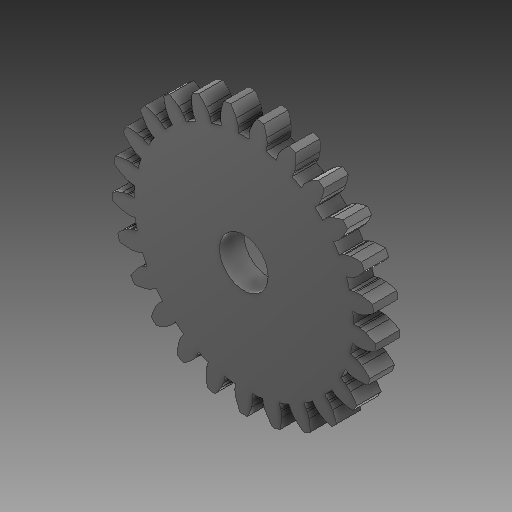
# Autodesk Inventor part: 歯車m2.z25
Saved by Autodesk Inventor 2020 (Build 240168000, 168)
## iProperties
Created: 2019-09-03
Part Number: 歯車m2.z25
Material: アセタール樹脂、黒
Document SubType Name: Modeling
Designer: 雪村
Density: 1.425 g/cm^3
Appearance: 滑らか - 黒
Mass: 7.88044 g
Surface Area: 64.9831 cm^2
Volume: 5.53013 cm^3
Description: ジュラコン 5t
Author: 雪村
Autodesk Inventor part; units mm, degrees
ref_plane "YZ Plane" through (0, 0, 0) normal (1, 0, 0) x (0, 1, 0)
ref_plane "XZ Plane" through (0, 0, 0) normal (0, 1, 0) x (-1, 0, 0)
ref_plane "XY Plane" through (0, 0, 0) normal (0, 0, 1) x (1, 0, 0)
sketch "スケッチ1" plane through (0, 0, 0) normal (0, 0, 1) x (1, 0, 0)
  arc A0 (1.1831, 23.814) -> (1.1255, 23.4653) centre (3.4046, 23.2682) ccw
  arc A1 (1.549, 24.9027) -> (1.1831, 23.814) centre (7.3031, 22.3628) ccw
  arc A2 (2.6687, 26.8678) -> (1.549, 24.9027) centre (11.5034, 20.532) ccw
  arc A3 (-4.7764, 23.36) -> (-4.7455, 23.008) centre (-2.4889, 23.3838) ccw
  arc A4 (-4.6927, 24.5056) -> (-4.7764, 23.36) centre (1.5122, 23.4765) ccw
  arc A5 (-4.0969, 26.6874) -> (-4.6927, 24.5056) centre (6.036, 22.7477) ccw
  arc A6 (-10.4358, 21.4383) -> (-10.3182, 21.105) centre (-8.226, 22.0302) ccw
  arc A7 (-10.6396, 22.5687) -> (-10.4358, 21.4383) centre (-4.3736, 23.115) ccw
  arc A8 (-10.605, 24.8301) -> (-10.6396, 22.5687) centre (0.1892, 23.5341) ccw
  arc A9 (-15.4394, 18.1695) -> (-15.2427, 17.876) centre (-13.4463, 19.2924) ccw
  arc A10 (-15.9179, 19.2137) -> (-15.4394, 18.1695) centre (-9.9847, 21.3011) ccw
  arc A11 (-16.4468, 21.4126) -> (-15.9179, 19.2137) centre (-5.6694, 22.8418) ccw
  arc A12 (-19.4729, 13.7591) -> (-19.2094, 13.5236) centre (-17.8217, 15.3423) ccw
  arc A13 (-20.1961, 14.6514) -> (-19.4729, 13.7591) centre (-14.9684, 18.1488) ccw
  arc A14 (-21.2552, 16.6498) -> (-20.1961, 14.6514) centre (-11.1719, 20.7143) ccw
  arc A15 (-22.2829, 8.4841) -> (-21.9691, 8.3216) centre (-21.0772, 10.4282) ccw
  arc A16 (-23.2052, 9.1685) -> (-22.2829, 8.4841) centre (-19.0115, 13.8562) ccw
  arc A17 (-24.7281, 10.8407) -> (-23.2052, 9.1685) centre (-15.9723, 17.2852) ccw
  arc A18 (-23.6927, 2.676) -> (-23.3484, 2.5967) centre (-23.0085, 4.8589) ccw
  arc A19 (-24.7563, 3.1096) -> (-23.6927, 2.676) centre (-21.8601, 8.6929) ccw
  arc A20 (-26.6472, 4.3505) -> (-24.7563, 3.1096) centre (-19.7691, 12.77) ccw
  arc A21 (-23.6139, -3.3002) -> (-23.2606, -3.2914) centre (-23.494, -1.0157) ccw
  arc A22 (-24.7519, -3.1447) -> (-23.6139, -3.3002) centre (-23.3352, 2.9834) ccw
  arc A23 (-26.892, -2.4131) -> (-24.7519, -3.1447) centre (-22.3238, 7.4524) ccw
  arc A24 (-22.0513, -9.069) -> (-21.7113, -8.9727) centre (-22.5033, -6.8265) ccw
  arc A25 (-23.1922, -9.2015) -> (-22.0513, -9.069) centre (-23.344, -2.9136) ccw
  arc A26 (-25.447, -9.025) -> (-23.1922, -9.2015) centre (-23.4758, 1.6665) ccw
  arc A27 (-19.1031, -14.268) -> (-18.7978, -14.0902) centre (-20.0986, -12.2084) ccw
  arc A28 (-20.1752, -14.6801) -> (-19.1031, -14.268) centre (-21.886, -8.6275) ccw
  arc A29 (-22.4031, -15.0699) -> (-20.1752, -14.6801) centre (-23.1527, -4.224) ccw
  arc A30 (-14.9546, -18.5705) -> (-14.7031, -18.3223) centre (-16.4311, -16.8231) ccw
  arc A31 (-15.8906, -19.2363) -> (-14.9546, -18.5705) centre (-19.0529, -13.7993) ccw
  arc A32 (-17.9515, -20.1679) -> (-15.8906, -19.2363) centre (-21.3749, -9.8492) ccw
  arc A33 (-9.8665, -21.7062) -> (-9.6846, -21.4032) centre (-11.7311, -20.3809) ccw
  arc A34 (-10.6075, -22.5837) -> (-9.8665, -21.7062) centre (-15.0226, -18.104) ccw
  arc A35 (-12.372, -23.9986) -> (-10.6075, -22.5837) centre (-18.254, -14.8554) ccw
  arc A36 (-4.1584, -23.4779) -> (-4.0576, -23.1392) centre (-6.294, -22.658) ccw
  arc A37 (-4.6579, -24.5122) -> (-4.1584, -23.4779) centre (-10.0483, -21.2712) ccw
  arc A38 (-6.0151, -26.3214) -> (-4.6579, -24.5122) centre (-13.9861, -18.9283) ccw
  arc A39 (1.811, -23.7745) -> (1.8244, -23.4214) centre (-0.4615, -23.5114) ccw
  arc A40 (1.5844, -24.9005) -> (1.811, -23.7745) centre (-4.4427, -23.1018) ccw
  arc A41 (0.7197, -26.9904) -> (1.5844, -24.9005) centre (-8.8394, -21.8118) ccw
  arc A42 (7.6665, -22.5772) -> (7.5917, -22.2318) centre (5.4, -22.8875) ccw
  arc A43 (7.7271, -23.7242) -> (7.6665, -22.5772) centre (1.4421, -23.4809) ccw
  arc A44 (7.4094, -25.9635) -> (7.7271, -23.7242) centre (-3.1373, -23.3248) ccw
  arc A45 (13.0404, -19.9613) -> (12.882, -19.6454) centre (10.9223, -20.8255) ccw
  arc A46 (13.3843, -21.0572) -> (13.0404, -19.9613) centre (7.2362, -22.3846) ccw
  arc A47 (13.6334, -23.3051) -> (13.3843, -21.0572) centre (2.7619, -23.3723) ccw
  arc A48 (17.5949, -16.0912) -> (17.3629, -15.8246) centre (15.7582, -17.455) ccw
  arc A49 (18.2005, -17.0671) -> (17.5949, -16.0912) centre (12.5757, -19.8817) ccw
  arc A50 (19.0009, -19.1825) -> (18.2005, -17.0671) centre (8.4876, -21.9511) ccw
  arc A51 (21.0438, -11.21) -> (20.7529, -11.0094) centre (19.604, -12.9877) ccw
  arc A52 (21.8731, -12.0046) -> (21.0438, -11.21) centre (17.125, -16.1297) ccw
  arc A53 (23.1744, -13.8545) -> (21.8731, -12.0046) centre (13.68, -19.1507) ccw
  arc A54 (23.1705, -5.6244) -> (22.8388, -5.5025) centre (22.2181, -7.7043) ccw
  arc A55 (24.1714, -6.1879) -> (23.1705, -5.6244) centre (20.5983, -11.3641) ccw
  arc A56 (25.8918, -7.656) -> (24.1714, -6.1879) centre (18.0128, -15.147) ccw
  arc A57 (23.8413, 0.3146) -> (23.4897, 0.3501) centre (23.436, -1.9369) ccw
  arc A58 (24.9508, 0.0177) -> (23.8413, 0.3146) centre (22.7773, -5.8845) ccw
  arc A59 (26.9823, -0.9764) -> (24.9508, 0.0177) centre (21.2138, -10.1915) ccw
  arc A60 (23.014, 6.2338) -> (22.6647, 6.1808) centre (23.1814, 3.9523) ccw
  arc A61 (24.1626, 6.2222) -> (23.014, 6.2338) centre (23.5251, -0.0352) ccw
  arc A62 (26.3775, 5.7645) -> (24.1626, 6.2222) centre (23.0818, -4.5957) ccw
  arc A63 (20.7407, 11.7613) -> (20.4155, 11.6231) centre (21.4702, 9.5931) ccw
  arc A64 (21.8561, 12.0357) -> (20.7407, 11.7613) centre (22.7948, 5.8164) ccw
  arc A65 (24.1152, 12.1432) -> (21.8561, 12.0357) centre (23.4996, 1.2889) ccw
  arc A66 (17.1642, 16.5498) -> (16.8836, 16.335) centre (18.41, 14.6311) ccw
  arc A67 (18.1763, 17.0929) -> (17.1642, 16.5498) centre (20.6321, 11.3025) ccw
  arc A68 (20.3377, 17.7589) -> (18.1763, 17.0929) centre (22.4408, 7.0925) ccw
  arc A69 (12.5092, 20.2984) -> (12.2908, 20.0206) centre (14.193, 18.7499) ccw
  arc A70 (13.3544, 21.0762) -> (12.5092, 20.2984) centre (17.1731, 16.0784) ccw
  arc A71 (15.2823, 22.2587) -> (13.3544, 21.0762) centre (19.9719, 12.4505) ccw
  arc A72 (7.0682, 22.7716) -> (6.9257, 22.4482) centre (9.0842, 21.6904) ccw
  arc A73 (7.6934, 23.7351) -> (7.0682, 22.7716) centre (12.6351, 19.8441) ccw
  arc A74 (9.2666, 25.36) -> (7.6934, 23.7351) centre (16.2481, 17.0261) ccw
  arc A75 (-1.1255, 23.4653) -> (-1.1831, 23.814) centre (-3.4046, 23.2682) ccw
  arc A76 (-1.1831, 23.814) -> (-1.549, 24.9027) centre (-7.3031, 22.3628) ccw
  arc A77 (-1.549, 24.9027) -> (-2.6687, 26.8678) centre (-11.5034, 20.532) ccw
  arc A78 (-6.9257, 22.4482) -> (-7.0682, 22.7716) centre (-9.0842, 21.6904) ccw
  arc A79 (-7.0682, 22.7716) -> (-7.6934, 23.7351) centre (-12.6351, 19.8441) ccw
  arc A80 (-7.6934, 23.7351) -> (-9.2666, 25.36) centre (-16.2481, 17.0261) ccw
  arc A81 (-12.2908, 20.0206) -> (-12.5092, 20.2984) centre (-14.193, 18.7499) ccw
  arc A82 (-12.5092, 20.2984) -> (-13.3544, 21.0762) centre (-17.1731, 16.0784) ccw
  arc A83 (-13.3544, 21.0762) -> (-15.2823, 22.2587) centre (-19.9719, 12.4505) ccw
  arc A84 (-16.8836, 16.335) -> (-17.1642, 16.5498) centre (-18.41, 14.6311) ccw
  arc A85 (-17.1642, 16.5498) -> (-18.1763, 17.0929) centre (-20.6321, 11.3025) ccw
  arc A86 (-18.1763, 17.0929) -> (-20.3377, 17.7589) centre (-22.4408, 7.0925) ccw
  arc A87 (-20.4155, 11.6231) -> (-20.7407, 11.7613) centre (-21.4702, 9.5931) ccw
  arc A88 (-20.7407, 11.7613) -> (-21.8561, 12.0357) centre (-22.7948, 5.8164) ccw
  arc A89 (-21.8561, 12.0357) -> (-24.1152, 12.1432) centre (-23.4996, 1.2889) ccw
  arc A90 (-22.6647, 6.1808) -> (-23.014, 6.2338) centre (-23.1814, 3.9523) ccw
  arc A91 (-23.014, 6.2338) -> (-24.1626, 6.2222) centre (-23.5251, -0.0352) ccw
  arc A92 (-24.1626, 6.2222) -> (-26.3775, 5.7645) centre (-23.0818, -4.5957) ccw
  arc A93 (-23.4897, 0.3501) -> (-23.8413, 0.3146) centre (-23.436, -1.9369) ccw
  arc A94 (-23.8413, 0.3146) -> (-24.9508, 0.0177) centre (-22.7773, -5.8845) ccw
  arc A95 (-24.9508, 0.0177) -> (-26.9823, -0.9764) centre (-21.2138, -10.1915) ccw
  arc A96 (-22.8388, -5.5025) -> (-23.1705, -5.6244) centre (-22.2181, -7.7043) ccw
  arc A97 (-23.1705, -5.6244) -> (-24.1714, -6.1879) centre (-20.5983, -11.3641) ccw
  arc A98 (-24.1714, -6.1879) -> (-25.8918, -7.656) centre (-18.0128, -15.147) ccw
  arc A99 (-20.7529, -11.0094) -> (-21.0438, -11.21) centre (-19.604, -12.9877) ccw
  arc A100 (-21.0438, -11.21) -> (-21.8731, -12.0046) centre (-17.125, -16.1297) ccw
  arc A101 (-21.8731, -12.0046) -> (-23.1744, -13.8545) centre (-13.68, -19.1507) ccw
  arc A102 (-17.3629, -15.8246) -> (-17.5949, -16.0912) centre (-15.7582, -17.455) ccw
  arc A103 (-17.5949, -16.0912) -> (-18.2005, -17.0671) centre (-12.5757, -19.8817) ccw
  arc A104 (-18.2005, -17.0671) -> (-19.0009, -19.1825) centre (-8.4876, -21.9511) ccw
  arc A105 (-12.882, -19.6454) -> (-13.0404, -19.9613) centre (-10.9223, -20.8255) ccw
  arc A106 (-13.0404, -19.9613) -> (-13.3843, -21.0572) centre (-7.2362, -22.3846) ccw
  arc A107 (-13.3843, -21.0572) -> (-13.6334, -23.3051) centre (-2.7619, -23.3723) ccw
  arc A108 (-7.5917, -22.2318) -> (-7.6665, -22.5772) centre (-5.4, -22.8875) ccw
  arc A109 (-7.6665, -22.5772) -> (-7.7271, -23.7242) centre (-1.4421, -23.4809) ccw
  arc A110 (-7.7271, -23.7242) -> (-7.4094, -25.9635) centre (3.1373, -23.3248) ccw
  arc A111 (-1.8244, -23.4214) -> (-1.811, -23.7745) centre (0.4615, -23.5114) ccw
  arc A112 (-1.811, -23.7745) -> (-1.5844, -24.9005) centre (4.4427, -23.1018) ccw
  arc A113 (-1.5844, -24.9005) -> (-0.7197, -26.9904) centre (8.8394, -21.8118) ccw
  arc A114 (4.0576, -23.1392) -> (4.1584, -23.4779) centre (6.294, -22.658) ccw
  arc A115 (4.1584, -23.4779) -> (4.6579, -24.5122) centre (10.0483, -21.2712) ccw
  arc A116 (4.6579, -24.5122) -> (6.0151, -26.3214) centre (13.9861, -18.9283) ccw
  arc A117 (9.6846, -21.4032) -> (9.8665, -21.7062) centre (11.7311, -20.3809) ccw
  arc A118 (9.8665, -21.7062) -> (10.6075, -22.5837) centre (15.0226, -18.104) ccw
  arc A119 (10.6075, -22.5837) -> (12.372, -23.9986) centre (18.254, -14.8554) ccw
  arc A120 (14.7031, -18.3223) -> (14.9546, -18.5705) centre (16.4311, -16.8231) ccw
  arc A121 (14.9546, -18.5705) -> (15.8906, -19.2363) centre (19.0529, -13.7993) ccw
  arc A122 (15.8906, -19.2363) -> (17.9515, -20.1679) centre (21.3749, -9.8492) ccw
  arc A123 (18.7978, -14.0902) -> (19.1031, -14.268) centre (20.0986, -12.2084) ccw
  arc A124 (19.1031, -14.268) -> (20.1752, -14.6801) centre (21.886, -8.6275) ccw
  arc A125 (20.1752, -14.6801) -> (22.4031, -15.0699) centre (23.1527, -4.224) ccw
  arc A126 (21.7113, -8.9727) -> (22.0513, -9.069) centre (22.5033, -6.8265) ccw
  arc A127 (22.0513, -9.069) -> (23.1922, -9.2015) centre (23.344, -2.9136) ccw
  arc A128 (23.1922, -9.2015) -> (25.447, -9.025) centre (23.4758, 1.6665) ccw
  arc A129 (23.2606, -3.2914) -> (23.6139, -3.3002) centre (23.494, -1.0157) ccw
  arc A130 (23.6139, -3.3002) -> (24.7519, -3.1447) centre (23.3352, 2.9834) ccw
  arc A131 (24.7519, -3.1447) -> (26.892, -2.4131) centre (22.3238, 7.4524) ccw
  arc A132 (23.3484, 2.5967) -> (23.6927, 2.676) centre (23.0085, 4.8589) ccw
  arc A133 (23.6927, 2.676) -> (24.7563, 3.1096) centre (21.8601, 8.6929) ccw
  arc A134 (24.7563, 3.1096) -> (26.6472, 4.3505) centre (19.7691, 12.77) ccw
  arc A135 (21.9691, 8.3216) -> (22.2829, 8.4841) centre (21.0772, 10.4282) ccw
  arc A136 (22.2829, 8.4841) -> (23.2052, 9.1685) centre (19.0115, 13.8562) ccw
  arc A137 (23.2052, 9.1685) -> (24.7281, 10.8407) centre (15.9723, 17.2852) ccw
  arc A138 (19.2094, 13.5236) -> (19.4729, 13.7591) centre (17.8217, 15.3423) ccw
  arc A139 (19.4729, 13.7591) -> (20.1961, 14.6514) centre (14.9684, 18.1488) ccw
  arc A140 (20.1961, 14.6514) -> (21.2552, 16.6498) centre (11.1719, 20.7143) ccw
  arc A141 (15.2427, 17.876) -> (15.4394, 18.1695) centre (13.4463, 19.2924) ccw
  arc A142 (15.4394, 18.1695) -> (15.9179, 19.2137) centre (9.9847, 21.3011) ccw
  arc A143 (15.9179, 19.2137) -> (16.4468, 21.4126) centre (5.6694, 22.8418) ccw
  arc A144 (10.3182, 21.105) -> (10.4358, 21.4383) centre (8.226, 22.0302) ccw
  arc A145 (10.4358, 21.4383) -> (10.6396, 22.5687) centre (4.3736, 23.115) ccw
  arc A146 (10.6396, 22.5687) -> (10.605, 24.8301) centre (-0.1892, 23.5341) ccw
  arc A147 (4.7455, 23.008) -> (4.7764, 23.36) centre (2.4889, 23.3838) ccw
  arc A148 (4.7764, 23.36) -> (4.6927, 24.5056) centre (-1.5122, 23.4765) ccw
  arc A149 (4.6927, 24.5056) -> (4.0969, 26.6874) centre (-6.036, 22.7477) ccw
  arc A150 (1.078, 22.4742) -> (-1.078, 22.4742) centre (0, 0) ccw
  arc A151 (-4.545, 22.0362) -> (-6.6332, 21.5) centre (0, 0) ccw
  arc A152 (-9.8824, 20.2136) -> (-11.7716, 19.175) centre (0, 0) ccw
  arc A153 (-14.5988, 17.1209) -> (-16.1704, 15.645) centre (0, 0) ccw
  arc A154 (-18.398, 12.9524) -> (-19.5532, 11.1321) centre (0, 0) ccw
  arc A155 (-21.0411, 7.9701) -> (-21.7073, 5.9197) centre (0, 0) ccw
  arc A156 (-22.3621, 2.487) -> (-22.4975, 0.3353) centre (0, 0) ccw
  arc A157 (-22.2781, -3.1524) -> (-21.8741, -5.2701) centre (0, 0) ccw
  arc A158 (-20.7942, -8.5937) -> (-19.8763, -10.5444) centre (0, 0) ccw
  arc A159 (-18.0038, -13.495) -> (-16.6295, -15.1561) centre (0, 0) ccw
  arc A160 (-14.0821, -17.5484) -> (-12.3379, -18.8156) centre (0, 0) ccw
  arc A161 (-9.2755, -20.4991) -> (-7.271, -21.2928) centre (0, 0) ccw
  arc A162 (-3.8862, -22.1618) -> (-1.7473, -22.4321) centre (0, 0) ccw
  arc A163 (1.7473, -22.4321) -> (3.8862, -22.1618) centre (0, 0) ccw
  arc A164 (7.271, -21.2928) -> (9.2755, -20.4991) centre (0, 0) ccw
  arc A165 (12.3379, -18.8156) -> (14.0821, -17.5484) centre (0, 0) ccw
  arc A166 (16.6295, -15.1561) -> (18.0038, -13.495) centre (0, 0) ccw
  arc A167 (19.8763, -10.5444) -> (20.7942, -8.5937) centre (0, 0) ccw
  arc A168 (21.8741, -5.2701) -> (22.2781, -3.1524) centre (0, 0) ccw
  arc A169 (22.4975, 0.3353) -> (22.3621, 2.487) centre (0, 0) ccw
  arc A170 (21.7073, 5.9197) -> (21.0411, 7.9701) centre (0, 0) ccw
  arc A171 (19.5532, 11.1321) -> (18.398, 12.9524) centre (0, 0) ccw
  arc A172 (16.1704, 15.645) -> (14.5988, 17.1209) centre (0, 0) ccw
  arc A173 (11.7716, 19.175) -> (9.8824, 20.2136) centre (0, 0) ccw
  arc A174 (6.6332, 21.5) -> (4.545, 22.0362) centre (0, 0) ccw
  arc A175 (-2.6687, 26.8678) -> (-4.0969, 26.6874) centre (0, 0) ccw
  arc A176 (-9.2666, 25.36) -> (-10.605, 24.8301) centre (0, 0) ccw
  arc A177 (-15.2823, 22.2587) -> (-16.4468, 21.4126) centre (0, 0) ccw
  arc A178 (-20.3377, 17.7589) -> (-21.2552, 16.6498) centre (0, 0) ccw
  arc A179 (-24.1152, 12.1432) -> (-24.7281, 10.8407) centre (0, 0) ccw
  arc A180 (-26.3775, 5.7645) -> (-26.6472, 4.3505) centre (0, 0) ccw
  arc A181 (-26.9823, -0.9764) -> (-26.892, -2.4131) centre (0, 0) ccw
  arc A182 (-25.8918, -7.656) -> (-25.447, -9.025) centre (0, 0) ccw
  arc A183 (-23.1744, -13.8545) -> (-22.4031, -15.0699) centre (0, 0) ccw
  arc A184 (-19.0009, -19.1825) -> (-17.9515, -20.1679) centre (0, 0) ccw
  arc A185 (-13.6334, -23.3051) -> (-12.372, -23.9986) centre (0, 0) ccw
  arc A186 (-7.4094, -25.9635) -> (-6.0151, -26.3214) centre (0, 0) ccw
  arc A187 (-0.7197, -26.9904) -> (0.7197, -26.9904) centre (0, 0) ccw
  arc A188 (6.0151, -26.3214) -> (7.4094, -25.9635) centre (0, 0) ccw
  arc A189 (12.372, -23.9986) -> (13.6334, -23.3051) centre (0, 0) ccw
  arc A190 (17.9515, -20.1679) -> (19.0009, -19.1825) centre (0, 0) ccw
  arc A191 (22.4031, -15.0699) -> (23.1744, -13.8545) centre (0, 0) ccw
  arc A192 (25.447, -9.025) -> (25.8918, -7.656) centre (0, 0) ccw
  arc A193 (26.892, -2.4131) -> (26.9823, -0.9764) centre (0, 0) ccw
  arc A194 (26.6472, 4.3505) -> (26.3775, 5.7645) centre (0, 0) ccw
  arc A195 (24.7281, 10.8407) -> (24.1152, 12.1432) centre (0, 0) ccw
  arc A196 (21.2552, 16.6498) -> (20.3377, 17.7589) centre (0, 0) ccw
  arc A197 (16.4468, 21.4126) -> (15.2823, 22.2587) centre (0, 0) ccw
  arc A198 (10.605, 24.8301) -> (9.2666, 25.36) centre (0, 0) ccw
  arc A199 (4.0969, 26.6874) -> (2.6687, 26.8678) centre (0, 0) ccw
  line L0 (1.078, 22.4742) -> (1.1255, 23.4653)
  line L1 (-4.545, 22.0362) -> (-4.7455, 23.008)
  line L2 (-9.8824, 20.2136) -> (-10.3182, 21.105)
  line L3 (-14.5988, 17.1209) -> (-15.2427, 17.876)
  line L4 (-18.398, 12.9524) -> (-19.2094, 13.5236)
  line L5 (-21.0411, 7.9701) -> (-21.9691, 8.3216)
  line L6 (-22.3621, 2.487) -> (-23.3484, 2.5967)
  line L7 (-22.2781, -3.1524) -> (-23.2606, -3.2914)
  line L8 (-20.7942, -8.5937) -> (-21.7113, -8.9727)
  line L9 (-18.0038, -13.495) -> (-18.7978, -14.0902)
  line L10 (-14.0821, -17.5484) -> (-14.7031, -18.3223)
  line L11 (-9.2755, -20.4991) -> (-9.6846, -21.4032)
  line L12 (-3.8862, -22.1618) -> (-4.0576, -23.1392)
  line L13 (1.7473, -22.4321) -> (1.8244, -23.4214)
  line L14 (7.271, -21.2928) -> (7.5917, -22.2318)
  line L15 (12.3379, -18.8156) -> (12.882, -19.6454)
  line L16 (16.6295, -15.1561) -> (17.3629, -15.8246)
  line L17 (19.8763, -10.5444) -> (20.7529, -11.0094)
  line L18 (21.8741, -5.2701) -> (22.8388, -5.5025)
  line L19 (22.4975, 0.3353) -> (23.4897, 0.3501)
  line L20 (21.7073, 5.9197) -> (22.6647, 6.1808)
  line L21 (19.5532, 11.1321) -> (20.4155, 11.6231)
  line L22 (16.1704, 15.645) -> (16.8836, 16.335)
  line L23 (11.7716, 19.175) -> (12.2908, 20.0206)
  line L24 (6.6332, 21.5) -> (6.9257, 22.4482)
  line L25 (-1.078, 22.4742) -> (-1.1255, 23.4653)
  line L26 (-6.6332, 21.5) -> (-6.9257, 22.4482)
  line L27 (-11.7716, 19.175) -> (-12.2908, 20.0206)
  line L28 (-16.1704, 15.645) -> (-16.8836, 16.335)
  line L29 (-19.5532, 11.1321) -> (-20.4155, 11.6231)
  line L30 (-21.7073, 5.9197) -> (-22.6647, 6.1808)
  line L31 (-22.4975, 0.3353) -> (-23.4897, 0.3501)
  line L32 (-21.8741, -5.2701) -> (-22.8388, -5.5025)
  line L33 (-19.8763, -10.5444) -> (-20.7529, -11.0094)
  line L34 (-16.6295, -15.1561) -> (-17.3629, -15.8246)
  line L35 (-12.3379, -18.8156) -> (-12.882, -19.6454)
  line L36 (-7.271, -21.2928) -> (-7.5917, -22.2318)
  line L37 (-1.7473, -22.4321) -> (-1.8244, -23.4214)
  line L38 (3.8862, -22.1618) -> (4.0576, -23.1392)
  line L39 (9.2755, -20.4991) -> (9.6846, -21.4032)
  line L40 (14.0821, -17.5484) -> (14.7031, -18.3223)
  line L41 (18.0038, -13.495) -> (18.7978, -14.0902)
  line L42 (20.7942, -8.5937) -> (21.7113, -8.9727)
  line L43 (22.2781, -3.1524) -> (23.2606, -3.2914)
  line L44 (22.3621, 2.487) -> (23.3484, 2.5967)
  line L45 (21.0411, 7.9701) -> (21.9691, 8.3216)
  line L46 (18.398, 12.9524) -> (19.2094, 13.5236)
  line L47 (14.5988, 17.1209) -> (15.2427, 17.876)
  line L48 (9.8824, 20.2136) -> (10.3182, 21.105)
  line L49 (4.545, 22.0362) -> (4.7455, 23.008)
  line L50 (-29, 0) -> (29, 0)
  line L51 (0, -29) -> (0, 29)
  line L52 (47, 27) -> (117, 27)
  line L53 (47, 19) -> (117, 19)
  line L54 (47, 11) -> (117, 11)
  line L55 (47, 3) -> (117, 3)
  line L56 (47, -5) -> (117, -5)
  line L57 (47, -13) -> (117, -13)
  line L58 (47, -21) -> (117, -21)
  line L59 (47, -29) -> (117, -29)
  line L60 (47, -37) -> (117, -37)
  line L61 (47, -45) -> (117, -45)
  line L62 (47, -53) -> (117, -53)
  line L63 (47, -61) -> (117, -61)
  line L64 (47, -69) -> (117, -69)
  line L65 (47, 27) -> (47, -69)
  line L66 (117, 27) -> (117, -69)
  line L67 (82, 19) -> (82, -69)
  point P0 (0, 0)
  point P1 (53, 21)
  point P2 (55.5, 13)
  point P3 (55.5, 5)
  point P4 (53, -3)
  point P5 (55.5, -11)
  point P6 (50.5, -19)
  point P7 (53, -27)
  point P8 (53, -35)
  point P9 (53, -43)
  point P10 (55.5, -51)
  point P11 (55.5, -59)
  point P12 (53, -67)
  point P13 (83, 13)
  point P14 (98, 5)
  point P15 (99.25, -3)
  point P16 (95.5, -11)
  point P17 (98, -19)
  point P18 (91.75, -27)
  point P19 (98, -35)
  point P20 (98, -43)
  point P21 (93, -51)
  point P22 (1, 42.5)
  point P23 (1, 36.5)
  point P24 (17.1875, 42.5)
  point P25 (19.3125, 36.5)
  constraints: 300 point on circle, 150 centre point, 132 end point, 14 horizontal, 2 horizontal alignment, 2 midpoint, 2 vertical, 859 other
extrude "押し出し1" add sketch "スケッチ1" along normal blind 5 contours A1 A2 A199 A149 A148 A147 L49 A174 L24 A72 A73 A74 A198 A146 A145 A144 L48 A173 L23 A69 A70 A71 A197 A143 A142 A141 L47 A172 L22 A66 A67 A68 A196 A140 A139 A138 L46 A171 L21 A63 A64 A65 A195 A137 A136 A135 L45 A170 L20 A60 A61 A62 A194 A134 A133 A132 L44 A169 L19 A57 A58 A59 L50 L51 A150 L0 A0 | L51 L50 A95 A94 A93 L31 A156 L6 A18 A19 A20 A180 A92 A91 A90 L30 A155 L5 A15 A16 A17 A179 A89 A88 A87 L29 A154 L4 A12 A13 A14 A178 A86 A85 A84 L28 A153 L3 A9 A10 A11 A177 A83 A82 A81 L27 A152 L2 A6 A7 A8 A176 A80 A79 A78 L26 A151 L1 A3 A4 A5 A175 A77 A76 A75 L25 A150 | L51 A187 A113 A112 A111 L37 A162 L12 A36 A37 A38 A186 A110 A109 A108 L36 A161 L11 A33 A34 A35 A185 A107 A106 A105 L35 A160 L10 A30 A31 A32 A184 A104 A103 A102 L34 A159 L9 A27 A28 A29 A183 A101 A100 A99 L33 A158 L8 A24 A25 A26 A182 A98 A97 A96 L32 A157 L7 A21 A22 A23 A181 A95 L50 | L50 A59 A193 A131 A130 A129 L43 A168 L18 A54 A55 A56 A192 A128 A127 A126 L42 A167 L17 A51 A52 A53 A191 A125 A124 A123 L41 A166 L16 A48 A49 A50 A190 A122 A121 A120 L40 A165 L15 A45 A46 A47 A189 A119 A118 A117 L39 A164 L14 A42 A43 A44 A188 A116 A115 A114 L38 A163 L13 A39 A40 A41 A187 L51
sketch "スケッチ2" plane through (0, 0, 5) normal (0, 0, 1) x (1, 0, 0)
  circle A0 centre (0, 0) radius 5
  dimension "d2" = 10
  constraints: 1 centre point, 1 coincident
  measures "d2" diameter of A0
extrude "押し出し2" cut sketch "スケッチ2" against normal through all
sketch "スケッチ3" plane through (0, 0, 5) normal (0, 0, 1) x (1, 0, 0)
  circle A0 centre (0, 0) radius 8
  circle A1 centre (0, 0) radius 5
  circle A2 centre (0, 0) radius 19.5
  line L0 (0, 15.6403) -> (0, -15.6403)
  line L1 (-15.4429, 0) -> (15.4429, 0)
  line L2 (-1, 19.4743) -> (-1.5, 7.8581)
  line L3 (1, 19.4743) -> (1.5, 7.8581)
  line L4 (7.8581, 1.5) -> (19.4743, 1)
  line L5 (7.8581, -1.5) -> (19.4743, -1)
  circle A3 centre (0, 0) radius 8
  line L6 (1.5, -7.8581) -> (1, -19.4743)
  line L7 (-19.4743, 1) -> (-7.8581, 1.5)
  line L8 (-19.4743, -1) -> (-7.8581, -1.5)
  line L9 (-1.5, -7.8581) -> (-1, -19.4743)
  circle A4 centre (0, 0) radius 5
  circle A5 centre (0, 0) radius 22.5
  circle A6 centre (0, 0) radius 5 projected
  point P0 (16.9761, 62.7038)
  point P1 (20.9761, 62.7038)
  point P2 (11.2302, 68.4498)
  point P3 (11.2302, 72.4498)
  point P4 (16.9761, 62.7038)
  point P5 (20.9761, 62.7038)
  point P6 (11.2302, 68.4498)
  point P7 (11.2302, 72.4498)
  point P8 (-9.8824, 20.2136)
  point P9 (-2, -7.746)
  point P10 (2, -7.746)
  point P11 (-7.746, -2)
  point P12 (-7.746, 2)
  point P13 (-9.8824, 20.2136)
  point P14 (-1.5, -7.8581)
  point P15 (-7.8581, -1.5)
  point P16 (1.5, -7.8581)
  point P17 (-7.8581, 1.5)
  dimension "d21" = 3
  dimension "d5" = 1
  dimension "d6" = 1
  dimension "d7" = 1
  dimension "d8" = 1
  dimension "d9" = 1
  dimension "d10" = 1
  dimension "d11" = 1
  dimension "d12" = 1
  dimension "d13" = 1.5
  dimension "d14" = 1.5
  dimension "d15" = 1.5
  dimension "d16" = 1.5
  dimension "d17" = 1.5
  dimension "d18" = 1.5
  dimension "d19" = 1.5
  dimension "d20" = 1.5
  dimension "d22" = 3
  constraints: 20 end point, 5 concentric, 4 point on circle, 3 centre point, 3 coincident, 2 midpoint, 1 horizontal, 1 vertical, 22 other
  measures "d5" distance from line of L0 L2.start
  measures "d6" distance from line of L3.start L0
  measures "d7" distance from line of L1 L4.end
  measures "d8" distance from line of L5.end L1
  measures "d9" distance from line of L0 L6.end
  measures "d10" distance from line of L0 L9.end
  measures "d11" distance from line of L1 L8.start
  measures "d12" distance from line of L1 L7.start
  measures "d13" distance from line of L0 L2.end
  measures "d14" distance from line of L0 L3.end
  measures "d15" distance from line of L1 L4.start
  measures "d16" distance from line of L5.start L1
  measures "d17" distance from line of L0 L6.start
  measures "d18" distance from line of L9.start L0
  measures "d19" distance from line of L1 L8.end
  measures "d20" distance from line of L1 L7.end
  measures "d22" radial gap between concentric circles of A0 A1
extrude "押し出し3" cut sketch "スケッチ3" against normal through all contours A0 L3 A2 L4 | L5 A2 L6 A0 | A0 L7 A2 L2 | L9 A2 L8 A0
fillet "フィレット1" radius 2 16 edges at (1, 19.4743, 2.5) (-1, 19.4743, 2.5) (-1.5, 7.8581, 2.5) (1.5, 7.8581, 2.5) (7.8581, -1.5, 2.5) (7.8581, 1.5, 2.5) (19.4743, 1, 2.5) (19.4743, -1, 2.5) (1.5, -7.8581, 2.5) (-1.5, -7.8581, 2.5) (-1, -19.4743, 2.5) (1, -19.4743, 2.5) (-7.8581, -1.5, 2.5) (-7.8581, 1.5, 2.5) (-19.4743, -1, 2.5) (-19.4743, 1, 2.5)
sketch "スケッチ4" plane through (0, 0, 5) normal (0, 0, 1) x (1, 0, 0)
  line L0 (9.3052, -1.4377) -> (17.1375, -1.1006) projected
  arc A0 (19.1919, -3.4529) -> (17.1375, -1.1006) centre (17.2235, -3.0987) ccw projected
  arc A1 (3.4529, -19.1919) -> (19.1919, -3.4529) centre (0, 0) ccw projected
  arc A2 (1.1006, -17.1375) -> (3.4529, -19.1919) centre (3.0987, -17.2235) ccw projected
  line L1 (1.1006, -17.1375) -> (1.4377, -9.3052) projected
  arc A3 (2.7487, -7.513) -> (1.4377, -9.3052) centre (3.4359, -9.3912) ccw projected
  arc A4 (2.7487, -7.513) -> (7.513, -2.7487) centre (0, 0) ccw projected
  arc A5 (9.3052, -1.4377) -> (7.513, -2.7487) centre (9.3912, -3.4359) ccw projected
  line L2 (1.4377, 9.3052) -> (1.1006, 17.1375) projected
  arc A6 (3.4529, 19.1919) -> (1.1006, 17.1375) centre (3.0987, 17.2235) ccw projected
  arc A7 (19.1919, 3.4529) -> (3.4529, 19.1919) centre (0, 0) ccw projected
  arc A8 (17.1375, 1.1006) -> (19.1919, 3.4529) centre (17.2235, 3.0987) ccw projected
  line L3 (17.1375, 1.1006) -> (9.3052, 1.4377) projected
  arc A9 (7.513, 2.7487) -> (9.3052, 1.4377) centre (9.3912, 3.4359) ccw projected
  arc A10 (7.513, 2.7487) -> (2.7487, 7.513) centre (0, 0) ccw projected
  arc A11 (1.4377, 9.3052) -> (2.7487, 7.513) centre (3.4359, 9.3912) ccw projected
  arc A12 (-7.513, -2.7487) -> (-2.7487, -7.513) centre (0, 0) ccw projected
  arc A13 (-1.4377, -9.3052) -> (-2.7487, -7.513) centre (-3.4359, -9.3912) ccw projected
  line L4 (-1.4377, -9.3052) -> (-1.1006, -17.1375) projected
  arc A14 (-3.4529, -19.1919) -> (-1.1006, -17.1375) centre (-3.0987, -17.2235) ccw projected
  arc A15 (-19.1919, -3.4529) -> (-3.4529, -19.1919) centre (0, 0) ccw projected
  arc A16 (-17.1375, -1.1006) -> (-19.1919, -3.4529) centre (-17.2235, -3.0987) ccw projected
  line L5 (-17.1375, -1.1006) -> (-9.3052, -1.4377) projected
  arc A17 (-7.513, -2.7487) -> (-9.3052, -1.4377) centre (-9.3912, -3.4359) ccw projected
  arc A18 (-3.4529, 19.1919) -> (-19.1919, 3.4529) centre (0, 0) ccw projected
  arc A19 (-1.1006, 17.1375) -> (-3.4529, 19.1919) centre (-3.0987, 17.2235) ccw projected
  line L6 (-1.1006, 17.1375) -> (-1.4377, 9.3052) projected
  arc A20 (-2.7487, 7.513) -> (-1.4377, 9.3052) centre (-3.4359, 9.3912) ccw projected
  arc A21 (-2.7487, 7.513) -> (-7.513, 2.7487) centre (0, 0) ccw projected
  arc A22 (-9.3052, 1.4377) -> (-7.513, 2.7487) centre (-9.3912, 3.4359) ccw projected
  line L7 (-9.3052, 1.4377) -> (-17.1375, 1.1006) projected
  arc A23 (-19.1919, 3.4529) -> (-17.1375, 1.1006) centre (-17.2235, 3.0987) ccw projected
  circle A24 centre (0, 0) radius 5 projected
  line L8 (18.0038, -13.495) -> (18.7978, -14.0902) projected
  arc A25 (18.7978, -14.0902) -> (19.1031, -14.268) centre (20.0986, -12.2084) ccw projected
  arc A26 (19.1031, -14.268) -> (20.1752, -14.6801) centre (21.886, -8.6275) ccw projected
  arc A27 (20.1752, -14.6801) -> (22.4031, -15.0699) centre (23.1527, -4.224) ccw projected
  arc A28 (22.4031, -15.0699) -> (23.1744, -13.8545) centre (0, 0) ccw projected
  arc A29 (23.1744, -13.8545) -> (21.8731, -12.0046) centre (13.68, -19.1507) ccw projected
  arc A30 (21.8731, -12.0046) -> (21.0438, -11.21) centre (17.125, -16.1297) ccw projected
  arc A31 (21.0438, -11.21) -> (20.7529, -11.0094) centre (19.604, -12.9877) ccw projected
  line L9 (20.7529, -11.0094) -> (19.8763, -10.5444) projected
  arc A32 (19.8763, -10.5444) -> (20.7942, -8.5937) centre (0, 0) ccw projected
  line L10 (20.7942, -8.5937) -> (21.7113, -8.9727) projected
  arc A33 (21.7113, -8.9727) -> (22.0513, -9.069) centre (22.5033, -6.8265) ccw projected
  arc A34 (22.0513, -9.069) -> (23.1922, -9.2015) centre (23.344, -2.9136) ccw projected
  arc A35 (23.1922, -9.2015) -> (25.447, -9.025) centre (23.4758, 1.6665) ccw projected
  arc A36 (25.447, -9.025) -> (25.8918, -7.656) centre (0, 0) ccw projected
  arc A37 (25.8918, -7.656) -> (24.1714, -6.1879) centre (18.0128, -15.147) ccw projected
  arc A38 (24.1714, -6.1879) -> (23.1705, -5.6244) centre (20.5983, -11.3641) ccw projected
  arc A39 (23.1705, -5.6244) -> (22.8388, -5.5025) centre (22.2181, -7.7043) ccw projected
  line L11 (22.8388, -5.5025) -> (21.8741, -5.2701) projected
  arc A40 (21.8741, -5.2701) -> (22.2781, -3.1524) centre (0, 0) ccw projected
  line L12 (22.2781, -3.1524) -> (23.2606, -3.2914) projected
  arc A41 (23.2606, -3.2914) -> (23.6139, -3.3002) centre (23.494, -1.0157) ccw projected
  arc A42 (23.6139, -3.3002) -> (24.7519, -3.1447) centre (23.3352, 2.9834) ccw projected
  arc A43 (24.7519, -3.1447) -> (26.892, -2.4131) centre (22.3238, 7.4524) ccw projected
  arc A44 (26.892, -2.4131) -> (26.9823, -0.9764) centre (0, 0) ccw projected
  arc A45 (26.9823, -0.9764) -> (24.9508, 0.0177) centre (21.2138, -10.1915) ccw projected
  arc A46 (24.9508, 0.0177) -> (23.8413, 0.3146) centre (22.7773, -5.8845) ccw projected
  arc A47 (23.8413, 0.3146) -> (23.4897, 0.3501) centre (23.436, -1.9369) ccw projected
  line L13 (23.4897, 0.3501) -> (22.4975, 0.3353) projected
  arc A48 (22.4975, 0.3353) -> (22.3621, 2.487) centre (0, 0) ccw projected
  line L14 (22.3621, 2.487) -> (23.3484, 2.5967) projected
  arc A49 (23.3484, 2.5967) -> (23.6927, 2.676) centre (23.0085, 4.8589) ccw projected
  arc A50 (23.6927, 2.676) -> (24.7563, 3.1096) centre (21.8601, 8.6929) ccw projected
  arc A51 (24.7563, 3.1096) -> (26.6472, 4.3505) centre (19.7691, 12.77) ccw projected
  arc A52 (26.6472, 4.3505) -> (26.3775, 5.7645) centre (0, 0) ccw projected
  arc A53 (26.3775, 5.7645) -> (24.1626, 6.2222) centre (23.0818, -4.5957) ccw projected
  arc A54 (24.1626, 6.2222) -> (23.014, 6.2338) centre (23.5251, -0.0352) ccw projected
  arc A55 (23.014, 6.2338) -> (22.6647, 6.1808) centre (23.1814, 3.9523) ccw projected
  line L15 (22.6647, 6.1808) -> (21.7073, 5.9197) projected
  arc A56 (21.7073, 5.9197) -> (21.0411, 7.9701) centre (0, 0) ccw projected
  line L16 (21.0411, 7.9701) -> (21.9691, 8.3216) projected
  arc A57 (21.9691, 8.3216) -> (22.2829, 8.4841) centre (21.0772, 10.4282) ccw projected
  arc A58 (22.2829, 8.4841) -> (23.2052, 9.1685) centre (19.0115, 13.8562) ccw projected
  arc A59 (23.2052, 9.1685) -> (24.7281, 10.8407) centre (15.9723, 17.2852) ccw projected
  arc A60 (24.7281, 10.8407) -> (24.1152, 12.1432) centre (0, 0) ccw projected
  arc A61 (24.1152, 12.1432) -> (21.8561, 12.0357) centre (23.4996, 1.2889) ccw projected
  arc A62 (21.8561, 12.0357) -> (20.7407, 11.7613) centre (22.7948, 5.8164) ccw projected
  arc A63 (20.7407, 11.7613) -> (20.4155, 11.6231) centre (21.4702, 9.5931) ccw projected
  line L17 (20.4155, 11.6231) -> (19.5532, 11.1321) projected
  arc A64 (19.5532, 11.1321) -> (18.398, 12.9524) centre (0, 0) ccw projected
  line L18 (18.398, 12.9524) -> (19.2094, 13.5236) projected
  arc A65 (19.2094, 13.5236) -> (19.4729, 13.7591) centre (17.8217, 15.3423) ccw projected
  arc A66 (19.4729, 13.7591) -> (20.1961, 14.6514) centre (14.9684, 18.1488) ccw projected
  arc A67 (20.1961, 14.6514) -> (21.2552, 16.6498) centre (11.1719, 20.7143) ccw projected
  arc A68 (21.2552, 16.6498) -> (20.3377, 17.7589) centre (0, 0) ccw projected
  arc A69 (20.3377, 17.7589) -> (18.1763, 17.0929) centre (22.4408, 7.0925) ccw projected
  arc A70 (18.1763, 17.0929) -> (17.1642, 16.5498) centre (20.6321, 11.3025) ccw projected
  arc A71 (17.1642, 16.5498) -> (16.8836, 16.335) centre (18.41, 14.6311) ccw projected
  line L19 (16.8836, 16.335) -> (16.1704, 15.645) projected
  arc A72 (16.1704, 15.645) -> (14.5988, 17.1209) centre (0, 0) ccw projected
  line L20 (14.5988, 17.1209) -> (15.2427, 17.876) projected
  arc A73 (15.2427, 17.876) -> (15.4394, 18.1695) centre (13.4463, 19.2924) ccw projected
  arc A74 (15.4394, 18.1695) -> (15.9179, 19.2137) centre (9.9847, 21.3011) ccw projected
  arc A75 (15.9179, 19.2137) -> (16.4468, 21.4126) centre (5.6694, 22.8418) ccw projected
  arc A76 (16.4468, 21.4126) -> (15.2823, 22.2587) centre (0, 0) ccw projected
  arc A77 (15.2823, 22.2587) -> (13.3544, 21.0762) centre (19.9719, 12.4505) ccw projected
  arc A78 (13.3544, 21.0762) -> (12.5092, 20.2984) centre (17.1731, 16.0784) ccw projected
  arc A79 (12.5092, 20.2984) -> (12.2908, 20.0206) centre (14.193, 18.7499) ccw projected
  line L21 (12.2908, 20.0206) -> (11.7716, 19.175) projected
  arc A80 (11.7716, 19.175) -> (9.8824, 20.2136) centre (0, 0) ccw projected
  line L22 (9.8824, 20.2136) -> (10.3182, 21.105) projected
  arc A81 (10.3182, 21.105) -> (10.4358, 21.4383) centre (8.226, 22.0302) ccw projected
  arc A82 (10.4358, 21.4383) -> (10.6396, 22.5687) centre (4.3736, 23.115) ccw projected
  arc A83 (10.6396, 22.5687) -> (10.605, 24.8301) centre (-0.1892, 23.5341) ccw projected
  arc A84 (10.605, 24.8301) -> (9.2666, 25.36) centre (0, 0) ccw projected
  arc A85 (9.2666, 25.36) -> (7.6934, 23.7351) centre (16.2481, 17.0261) ccw projected
  arc A86 (7.6934, 23.7351) -> (7.0682, 22.7716) centre (12.6351, 19.8441) ccw projected
  arc A87 (7.0682, 22.7716) -> (6.9257, 22.4482) centre (9.0842, 21.6904) ccw projected
  line L23 (6.9257, 22.4482) -> (6.6332, 21.5) projected
  arc A88 (6.6332, 21.5) -> (4.545, 22.0362) centre (0, 0) ccw projected
  line L24 (4.545, 22.0362) -> (4.7455, 23.008) projected
  arc A89 (4.7455, 23.008) -> (4.7764, 23.36) centre (2.4889, 23.3838) ccw projected
  arc A90 (4.7764, 23.36) -> (4.6927, 24.5056) centre (-1.5122, 23.4765) ccw projected
  arc A91 (4.6927, 24.5056) -> (4.0969, 26.6874) centre (-6.036, 22.7477) ccw projected
  arc A92 (4.0969, 26.6874) -> (2.6687, 26.8678) centre (0, 0) ccw projected
  arc A93 (2.6687, 26.8678) -> (1.549, 24.9027) centre (11.5034, 20.532) ccw projected
  arc A94 (1.549, 24.9027) -> (1.1831, 23.814) centre (7.3031, 22.3628) ccw projected
  arc A95 (1.1831, 23.814) -> (1.1255, 23.4653) centre (3.4046, 23.2682) ccw projected
  line L25 (1.1255, 23.4653) -> (1.078, 22.4742) projected
  arc A96 (1.078, 22.4742) -> (-1.078, 22.4742) centre (0, 0) ccw projected
  line L26 (-1.078, 22.4742) -> (-1.1255, 23.4653) projected
  arc A97 (-1.1255, 23.4653) -> (-1.1831, 23.814) centre (-3.4046, 23.2682) ccw projected
  arc A98 (-1.1831, 23.814) -> (-1.549, 24.9027) centre (-7.3031, 22.3628) ccw projected
  arc A99 (-1.549, 24.9027) -> (-2.6687, 26.8678) centre (-11.5034, 20.532) ccw projected
  arc A100 (-2.6687, 26.8678) -> (-4.0969, 26.6874) centre (0, 0) ccw projected
  arc A101 (-4.0969, 26.6874) -> (-4.6927, 24.5056) centre (6.036, 22.7477) ccw projected
  arc A102 (-4.6927, 24.5056) -> (-4.7764, 23.36) centre (1.5122, 23.4765) ccw projected
  arc A103 (-4.7764, 23.36) -> (-4.7455, 23.008) centre (-2.4889, 23.3838) ccw projected
  line L27 (-4.7455, 23.008) -> (-4.545, 22.0362) projected
  arc A104 (-4.545, 22.0362) -> (-6.6332, 21.5) centre (0, 0) ccw projected
  line L28 (-6.6332, 21.5) -> (-6.9257, 22.4482) projected
  arc A105 (-6.9257, 22.4482) -> (-7.0682, 22.7716) centre (-9.0842, 21.6904) ccw projected
  arc A106 (-7.0682, 22.7716) -> (-7.6934, 23.7351) centre (-12.6351, 19.8441) ccw projected
  arc A107 (-7.6934, 23.7351) -> (-9.2666, 25.36) centre (-16.2481, 17.0261) ccw projected
  arc A108 (-9.2666, 25.36) -> (-10.605, 24.8301) centre (0, 0) ccw projected
  arc A109 (-10.605, 24.8301) -> (-10.6396, 22.5687) centre (0.1892, 23.5341) ccw projected
  arc A110 (-10.6396, 22.5687) -> (-10.4358, 21.4383) centre (-4.3736, 23.115) ccw projected
  arc A111 (-10.4358, 21.4383) -> (-10.3182, 21.105) centre (-8.226, 22.0302) ccw projected
  line L29 (-10.3182, 21.105) -> (-9.8824, 20.2136) projected
  arc A112 (-9.8824, 20.2136) -> (-11.7716, 19.175) centre (0, 0) ccw projected
  line L30 (-11.7716, 19.175) -> (-12.2908, 20.0206) projected
  arc A113 (-12.2908, 20.0206) -> (-12.5092, 20.2984) centre (-14.193, 18.7499) ccw projected
  arc A114 (-12.5092, 20.2984) -> (-13.3544, 21.0762) centre (-17.1731, 16.0784) ccw projected
  arc A115 (-13.3544, 21.0762) -> (-15.2823, 22.2587) centre (-19.9719, 12.4505) ccw projected
  arc A116 (-15.2823, 22.2587) -> (-16.4468, 21.4126) centre (0, 0) ccw projected
  arc A117 (-16.4468, 21.4126) -> (-15.9179, 19.2137) centre (-5.6694, 22.8418) ccw projected
  arc A118 (-15.9179, 19.2137) -> (-15.4394, 18.1695) centre (-9.9847, 21.3011) ccw projected
  arc A119 (-15.4394, 18.1695) -> (-15.2427, 17.876) centre (-13.4463, 19.2924) ccw projected
  line L31 (-15.2427, 17.876) -> (-14.5988, 17.1209) projected
  arc A120 (-14.5988, 17.1209) -> (-16.1704, 15.645) centre (0, 0) ccw projected
  line L32 (-16.1704, 15.645) -> (-16.8836, 16.335) projected
  arc A121 (-16.8836, 16.335) -> (-17.1642, 16.5498) centre (-18.41, 14.6311) ccw projected
  arc A122 (-17.1642, 16.5498) -> (-18.1763, 17.0929) centre (-20.6321, 11.3025) ccw projected
  arc A123 (-18.1763, 17.0929) -> (-20.3377, 17.7589) centre (-22.4408, 7.0925) ccw projected
  arc A124 (-20.3377, 17.7589) -> (-21.2552, 16.6498) centre (0, 0) ccw projected
  arc A125 (-21.2552, 16.6498) -> (-20.1961, 14.6514) centre (-11.1719, 20.7143) ccw projected
  arc A126 (-20.1961, 14.6514) -> (-19.4729, 13.7591) centre (-14.9684, 18.1488) ccw projected
  arc A127 (-19.4729, 13.7591) -> (-19.2094, 13.5236) centre (-17.8217, 15.3423) ccw projected
  line L33 (-19.2094, 13.5236) -> (-18.398, 12.9524) projected
  arc A128 (-18.398, 12.9524) -> (-19.5532, 11.1321) centre (0, 0) ccw projected
  line L34 (-19.5532, 11.1321) -> (-20.4155, 11.6231) projected
  arc A129 (-20.4155, 11.6231) -> (-20.7407, 11.7613) centre (-21.4702, 9.5931) ccw projected
  arc A130 (-20.7407, 11.7613) -> (-21.8561, 12.0357) centre (-22.7948, 5.8164) ccw projected
  arc A131 (-21.8561, 12.0357) -> (-24.1152, 12.1432) centre (-23.4996, 1.2889) ccw projected
  arc A132 (-24.1152, 12.1432) -> (-24.7281, 10.8407) centre (0, 0) ccw projected
  arc A133 (-24.7281, 10.8407) -> (-23.2052, 9.1685) centre (-15.9723, 17.2852) ccw projected
  arc A134 (-23.2052, 9.1685) -> (-22.2829, 8.4841) centre (-19.0115, 13.8562) ccw projected
  arc A135 (-22.2829, 8.4841) -> (-21.9691, 8.3216) centre (-21.0772, 10.4282) ccw projected
  line L35 (-21.9691, 8.3216) -> (-21.0411, 7.9701) projected
  arc A136 (-21.0411, 7.9701) -> (-21.7073, 5.9197) centre (0, 0) ccw projected
  line L36 (-21.7073, 5.9197) -> (-22.6647, 6.1808) projected
  arc A137 (-22.6647, 6.1808) -> (-23.014, 6.2338) centre (-23.1814, 3.9523) ccw projected
  arc A138 (-23.014, 6.2338) -> (-24.1626, 6.2222) centre (-23.5251, -0.0352) ccw projected
  arc A139 (-24.1626, 6.2222) -> (-26.3775, 5.7645) centre (-23.0818, -4.5957) ccw projected
  arc A140 (-26.3775, 5.7645) -> (-26.6472, 4.3505) centre (0, 0) ccw projected
  arc A141 (-26.6472, 4.3505) -> (-24.7563, 3.1096) centre (-19.7691, 12.77) ccw projected
  arc A142 (-24.7563, 3.1096) -> (-23.6927, 2.676) centre (-21.8601, 8.6929) ccw projected
  arc A143 (-23.6927, 2.676) -> (-23.3484, 2.5967) centre (-23.0085, 4.8589) ccw projected
  line L37 (-23.3484, 2.5967) -> (-22.3621, 2.487) projected
  arc A144 (-22.3621, 2.487) -> (-22.4975, 0.3353) centre (0, 0) ccw projected
  line L38 (-22.4975, 0.3353) -> (-23.4897, 0.3501) projected
  arc A145 (-23.4897, 0.3501) -> (-23.8413, 0.3146) centre (-23.436, -1.9369) ccw projected
  arc A146 (-23.8413, 0.3146) -> (-24.9508, 0.0177) centre (-22.7773, -5.8845) ccw projected
  arc A147 (-24.9508, 0.0177) -> (-26.9823, -0.9764) centre (-21.2138, -10.1915) ccw projected
  arc A148 (-26.9823, -0.9764) -> (-26.892, -2.4131) centre (0, 0) ccw projected
  arc A149 (-26.892, -2.4131) -> (-24.7519, -3.1447) centre (-22.3238, 7.4524) ccw projected
  arc A150 (-24.7519, -3.1447) -> (-23.6139, -3.3002) centre (-23.3352, 2.9834) ccw projected
  arc A151 (-23.6139, -3.3002) -> (-23.2606, -3.2914) centre (-23.494, -1.0157) ccw projected
  line L39 (-23.2606, -3.2914) -> (-22.2781, -3.1524) projected
  arc A152 (-22.2781, -3.1524) -> (-21.8741, -5.2701) centre (0, 0) ccw projected
  line L40 (-21.8741, -5.2701) -> (-22.8388, -5.5025) projected
  arc A153 (-22.8388, -5.5025) -> (-23.1705, -5.6244) centre (-22.2181, -7.7043) ccw projected
  arc A154 (-23.1705, -5.6244) -> (-24.1714, -6.1879) centre (-20.5983, -11.3641) ccw projected
  arc A155 (-24.1714, -6.1879) -> (-25.8918, -7.656) centre (-18.0128, -15.147) ccw projected
  arc A156 (-25.8918, -7.656) -> (-25.447, -9.025) centre (0, 0) ccw projected
  arc A157 (-25.447, -9.025) -> (-23.1922, -9.2015) centre (-23.4758, 1.6665) ccw projected
  arc A158 (-23.1922, -9.2015) -> (-22.0513, -9.069) centre (-23.344, -2.9136) ccw projected
  arc A159 (-22.0513, -9.069) -> (-21.7113, -8.9727) centre (-22.5033, -6.8265) ccw projected
  line L41 (-21.7113, -8.9727) -> (-20.7942, -8.5937) projected
  arc A160 (-20.7942, -8.5937) -> (-19.8763, -10.5444) centre (0, 0) ccw projected
  line L42 (-19.8763, -10.5444) -> (-20.7529, -11.0094) projected
  arc A161 (-20.7529, -11.0094) -> (-21.0438, -11.21) centre (-19.604, -12.9877) ccw projected
  arc A162 (-21.0438, -11.21) -> (-21.8731, -12.0046) centre (-17.125, -16.1297) ccw projected
  arc A163 (-21.8731, -12.0046) -> (-23.1744, -13.8545) centre (-13.68, -19.1507) ccw projected
  arc A164 (-23.1744, -13.8545) -> (-22.4031, -15.0699) centre (0, 0) ccw projected
  arc A165 (-22.4031, -15.0699) -> (-20.1752, -14.6801) centre (-23.1527, -4.224) ccw projected
  arc A166 (-20.1752, -14.6801) -> (-19.1031, -14.268) centre (-21.886, -8.6275) ccw projected
  arc A167 (-19.1031, -14.268) -> (-18.7978, -14.0902) centre (-20.0986, -12.2084) ccw projected
  line L43 (-18.7978, -14.0902) -> (-18.0038, -13.495) projected
  arc A168 (-18.0038, -13.495) -> (-16.6295, -15.1561) centre (0, 0) ccw projected
  line L44 (-16.6295, -15.1561) -> (-17.3629, -15.8246) projected
  arc A169 (-17.3629, -15.8246) -> (-17.5949, -16.0912) centre (-15.7582, -17.455) ccw projected
  arc A170 (-17.5949, -16.0912) -> (-18.2005, -17.0671) centre (-12.5757, -19.8817) ccw projected
  arc A171 (-18.2005, -17.0671) -> (-19.0009, -19.1825) centre (-8.4876, -21.9511) ccw projected
  arc A172 (-19.0009, -19.1825) -> (-17.9515, -20.1679) centre (0, 0) ccw projected
  arc A173 (-17.9515, -20.1679) -> (-15.8906, -19.2363) centre (-21.3749, -9.8492) ccw projected
  arc A174 (-15.8906, -19.2363) -> (-14.9546, -18.5705) centre (-19.0529, -13.7993) ccw projected
  arc A175 (-14.9546, -18.5705) -> (-14.7031, -18.3223) centre (-16.4311, -16.8231) ccw projected
  line L45 (-14.7031, -18.3223) -> (-14.0821, -17.5484) projected
  arc A176 (-14.0821, -17.5484) -> (-12.3379, -18.8156) centre (0, 0) ccw projected
  line L46 (-12.3379, -18.8156) -> (-12.882, -19.6454) projected
  arc A177 (-12.882, -19.6454) -> (-13.0404, -19.9613) centre (-10.9223, -20.8255) ccw projected
  arc A178 (-13.0404, -19.9613) -> (-13.3843, -21.0572) centre (-7.2362, -22.3846) ccw projected
  arc A179 (-13.3843, -21.0572) -> (-13.6334, -23.3051) centre (-2.7619, -23.3723) ccw projected
  arc A180 (-13.6334, -23.3051) -> (-12.372, -23.9986) centre (0, 0) ccw projected
  arc A181 (-12.372, -23.9986) -> (-10.6075, -22.5837) centre (-18.254, -14.8554) ccw projected
  arc A182 (-10.6075, -22.5837) -> (-9.8665, -21.7062) centre (-15.0226, -18.104) ccw projected
  arc A183 (-9.8665, -21.7062) -> (-9.6846, -21.4032) centre (-11.7311, -20.3809) ccw projected
  line L47 (-9.6846, -21.4032) -> (-9.2755, -20.4991) projected
  arc A184 (-9.2755, -20.4991) -> (-7.271, -21.2928) centre (0, 0) ccw projected
  line L48 (-7.271, -21.2928) -> (-7.5917, -22.2318) projected
  arc A185 (-7.5917, -22.2318) -> (-7.6665, -22.5772) centre (-5.4, -22.8875) ccw projected
  arc A186 (-7.6665, -22.5772) -> (-7.7271, -23.7242) centre (-1.4421, -23.4809) ccw projected
  arc A187 (-7.7271, -23.7242) -> (-7.4094, -25.9635) centre (3.1373, -23.3248) ccw projected
  arc A188 (-7.4094, -25.9635) -> (-6.0151, -26.3214) centre (0, 0) ccw projected
  arc A189 (-6.0151, -26.3214) -> (-4.6579, -24.5122) centre (-13.9861, -18.9283) ccw projected
  arc A190 (-4.6579, -24.5122) -> (-4.1584, -23.4779) centre (-10.0483, -21.2712) ccw projected
  arc A191 (-4.1584, -23.4779) -> (-4.0576, -23.1392) centre (-6.294, -22.658) ccw projected
  line L49 (-4.0576, -23.1392) -> (-3.8862, -22.1618) projected
  arc A192 (-3.8862, -22.1618) -> (-1.7473, -22.4321) centre (0, 0) ccw projected
  line L50 (-1.7473, -22.4321) -> (-1.8244, -23.4214) projected
  arc A193 (-1.8244, -23.4214) -> (-1.811, -23.7745) centre (0.4615, -23.5114) ccw projected
  arc A194 (-1.811, -23.7745) -> (-1.5844, -24.9005) centre (4.4427, -23.1018) ccw projected
  arc A195 (-1.5844, -24.9005) -> (-0.7197, -26.9904) centre (8.8394, -21.8118) ccw projected
  arc A196 (-0.7197, -26.9904) -> (0.7197, -26.9904) centre (0, 0) ccw projected
  arc A197 (0.7197, -26.9904) -> (1.5844, -24.9005) centre (-8.8394, -21.8118) ccw projected
  arc A198 (1.5844, -24.9005) -> (1.811, -23.7745) centre (-4.4427, -23.1018) ccw projected
  arc A199 (1.811, -23.7745) -> (1.8244, -23.4214) centre (-0.4615, -23.5114) ccw projected
  line L51 (1.8244, -23.4214) -> (1.7473, -22.4321) projected
  arc A200 (1.7473, -22.4321) -> (3.8862, -22.1618) centre (0, 0) ccw projected
  line L52 (3.8862, -22.1618) -> (4.0576, -23.1392) projected
  arc A201 (4.0576, -23.1392) -> (4.1584, -23.4779) centre (6.294, -22.658) ccw projected
  arc A202 (4.1584, -23.4779) -> (4.6579, -24.5122) centre (10.0483, -21.2712) ccw projected
  arc A203 (4.6579, -24.5122) -> (6.0151, -26.3214) centre (13.9861, -18.9283) ccw projected
  arc A204 (6.0151, -26.3214) -> (7.4094, -25.9635) centre (0, 0) ccw projected
  arc A205 (7.4094, -25.9635) -> (7.7271, -23.7242) centre (-3.1373, -23.3248) ccw projected
  arc A206 (7.7271, -23.7242) -> (7.6665, -22.5772) centre (1.4421, -23.4809) ccw projected
  arc A207 (7.6665, -22.5772) -> (7.5917, -22.2318) centre (5.4, -22.8875) ccw projected
  line L53 (7.5917, -22.2318) -> (7.271, -21.2928) projected
  arc A208 (7.271, -21.2928) -> (9.2755, -20.4991) centre (0, 0) ccw projected
  line L54 (9.2755, -20.4991) -> (9.6846, -21.4032) projected
  arc A209 (9.6846, -21.4032) -> (9.8665, -21.7062) centre (11.7311, -20.3809) ccw projected
  arc A210 (9.8665, -21.7062) -> (10.6075, -22.5837) centre (15.0226, -18.104) ccw projected
  arc A211 (10.6075, -22.5837) -> (12.372, -23.9986) centre (18.254, -14.8554) ccw projected
  arc A212 (12.372, -23.9986) -> (13.6334, -23.3051) centre (0, 0) ccw projected
  arc A213 (13.6334, -23.3051) -> (13.3843, -21.0572) centre (2.7619, -23.3723) ccw projected
  arc A214 (13.3843, -21.0572) -> (13.0404, -19.9613) centre (7.2362, -22.3846) ccw projected
  arc A215 (13.0404, -19.9613) -> (12.882, -19.6454) centre (10.9223, -20.8255) ccw projected
  line L55 (12.882, -19.6454) -> (12.3379, -18.8156) projected
  arc A216 (12.3379, -18.8156) -> (14.0821, -17.5484) centre (0, 0) ccw projected
  line L56 (14.0821, -17.5484) -> (14.7031, -18.3223) projected
  arc A217 (14.7031, -18.3223) -> (14.9546, -18.5705) centre (16.4311, -16.8231) ccw projected
  arc A218 (14.9546, -18.5705) -> (15.8906, -19.2363) centre (19.0529, -13.7993) ccw projected
  arc A219 (15.8906, -19.2363) -> (17.9515, -20.1679) centre (21.3749, -9.8492) ccw projected
  arc A220 (17.9515, -20.1679) -> (19.0009, -19.1825) centre (0, 0) ccw projected
  arc A221 (19.0009, -19.1825) -> (18.2005, -17.0671) centre (8.4876, -21.9511) ccw projected
  arc A222 (18.2005, -17.0671) -> (17.5949, -16.0912) centre (12.5757, -19.8817) ccw projected
  arc A223 (17.5949, -16.0912) -> (17.3629, -15.8246) centre (15.7582, -17.455) ccw projected
  line L57 (17.3629, -15.8246) -> (16.6295, -15.1561) projected
  arc A224 (16.6295, -15.1561) -> (18.0038, -13.495) centre (0, 0) ccw projected
extrude "押し出し4" add sketch "スケッチ4" against normal blind 0.7 contours L0 A0 A1 A2 L1 A3 A4 A5 | L2 A6 A7 A8 L3 A9 A10 A11 | A12 A13 L4 A14 A15 A16 L5 A17 | A19 L6 A20 A21 A22 L7 A23 A18
equation "\"d6\" = d5"
equation "\"d7\" = d6"
equation "\"d8\" = d7"
equation "\"d9\" = d8"
equation "\"d10\" = d9"
equation "\"d11\" = d6"
equation "\"d12\" = d5"
equation "\"d14\" = d13"
equation "\"d15\" = d14"
equation "\"d16\" = d15"
equation "\"d17\" = d16"
equation "\"d18\" = d16"
equation "\"d19\" = d13"
equation "\"d20\" = d19"
